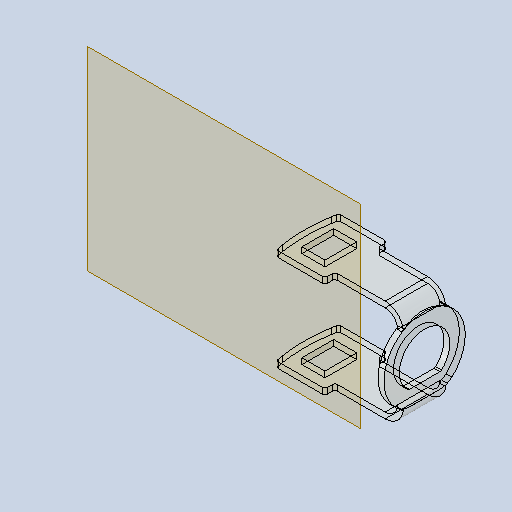
# Autodesk Inventor part: Part3 - Gearbox
Saved by Autodesk Inventor 2023 (Build 270158000, 158)
## iProperties
Created: 2020-10-26
Part Number: Part3 - Gearbox
Material: Glass
Document SubType Name: Modeling
Designer: Niels
Density: 2.18 g/cm^3
Appearance: Clear
MAAT: ØLxBxD
Author: Niels
Autodesk Inventor part; units mm, degrees
ref_plane "YZ Plane" through (0, 0, 0) normal (1, 0, 0) x (0, 1, 0)
ref_plane "XZ Plane" through (0, 0, 0) normal (0, 1, 0) x (-1, 0, 0)
ref_plane "XY Plane" through (0, 0, 0) normal (0, 0, 1) x (1, 0, 0)
ref_plane "Work Plane1" through (0, 0, -6) normal (0, 0, 1) x (1, 0, 0)
sketch "Sketch2" plane through (0, 0, -6) normal (0, 0, 1) x (1, 0, 0)
  line L0 (-0.1721, 1.3319) -> (-0.1721, -0.6681) projected
  line L1 (-0.1721, -0.6681) -> (-1.1721, -0.6681) projected
  line L2 (-1.1721, -0.6681) -> (-1.1721, -1.1681) projected
  line L3 (-1.1721, -1.1681) -> (0.1026, -1.1681) projected
  line L4 (0.1026, -1.1681) -> (1.1279, 1.3319) projected
  line L5 (-0.1721, 1.3319) -> (1.1279, 1.3319) projected
  line L6 (21.2279, 14.4069) -> (21.2279, 6.7069) projected
  line L7 (22.1279, 8.9819) -> (22.1279, 10.9819) projected
  line L8 (-1.5666, 1.1673) -> (16.9443, 1.1673)
  arc A0 (16.9443, 1.1673) -> (19.3523, 3.5752) centre (16.9443, 3.5752) ccw
  line L9 (19.3523, 3.5752) -> (19.3523, 9.9819)
  line L10 (20.5023, 9.9819) -> (20.5023, 3.5752)
  arc A1 (16.9443, 0.0173) -> (20.5023, 3.5752) centre (16.9443, 3.5752) ccw
  line L11 (16.9443, 0.0173) -> (-1.5666, 0.0173)
  line L12 (-1.5666, 0.0173) -> (-1.5666, 1.1673)
  line L13 (20.5023, 9.9819) -> (19.3523, 9.9819)
  line L14 (-1.5666, 18.7964) -> (16.9443, 18.7964)
  arc A2 (19.3523, 16.3885) -> (16.9443, 18.7964) centre (16.9443, 16.3885) ccw
  line L15 (19.3523, 16.3885) -> (19.3523, 9.9819)
  line L16 (20.5023, 9.9819) -> (20.5023, 16.3885)
  arc A3 (20.5023, 16.3885) -> (16.9443, 19.9464) centre (16.9443, 16.3885) ccw
  line L17 (16.9443, 19.9464) -> (-1.5666, 19.9464)
  line L18 (-1.5666, 19.9464) -> (-1.5666, 18.7964)
  point P0 (0, 0)
  point P1 (22.1279, 9.9819)
  dimension "d1" = 1.15
  dimension "d2" = 0.7257
  constraints: 22 end point, 8 point on circle, 7 symmetric about line, 4 centre point, 2 horizontal, 2 tangent, 1 horizontal alignment, 1 midpoint, 1 parallel, 1 vertical, 4 other
  measures "d1" radial gap between concentric circles of A0 A1
  measures "d2" distance between parallel lines of L6 L10
extrude "Extrusion1" add sketch "Sketch2" along normal mid plane 8.3 contours L8 L4 L11 L0 | L0 L11 L12 L8 | L8 A0 L9 L13 L10 A1 L11 L4 | L15 A2 L14 L18 L17 A3 L16 L13
sketch "Sketch3" plane through (20.5023, 3.5752, -1.85) normal (1, 0, 0) x (0, 0, -1)
  line L0 (1.1743, 2.6316) -> (7.1257, 2.6316) projected
  line L1 (1.1743, 2.6316) -> (7.1257, 2.6316) projected
  arc A0 (0.838, 2.7615) -> (1.1743, 2.6316) centre (1.1743, 3.1316) ccw projected
  arc A1 (7.462, 2.7615) -> (0.838, 2.7615) centre (4.15, 6.4066) ccw projected
  arc A2 (7.1257, 2.6316) -> (7.462, 2.7615) centre (7.1257, 3.1316) ccw projected
  line L2 (1.1743, 2.6316) -> (7.1257, 2.6316) projected
  arc A3 (-1.1794, 0.5412) -> (1.1743, -0.3684) centre (1.1743, 3.1316) ccw
  arc A4 (9.4794, 0.5412) -> (-1.1794, 0.5412) centre (4.15, 6.4066) ccw
  arc A5 (7.1257, -0.3684) -> (9.4794, 0.5412) centre (7.1257, 3.1316) ccw
  line L3 (7.1257, -0.3684) -> (1.1743, -0.3684)
  point P0 (-1.85, -3.5752)
  dimension "d5" = 3
  constraints: 6 point on circle, 3 centre point, 2 end point, 1 horizontal, 2 other
  measures "d5" radial gap between concentric circles of A1 A4
extrude "Extrusion2" add sketch "Sketch3" against normal blind 1.15
sketch "Sketch4" plane through (20.5023, 9.9819, -6) normal (1, 0, 0) x (0, 0, -1)
  line L0 (-2.9757, -3.775) -> (2.9757, -3.775) projected
  line L1 (-2.9757, -3.775) -> (2.9757, -3.775) projected
  arc A0 (-3.312, -3.6451) -> (-2.9757, -3.775) centre (-2.9757, -3.275) ccw projected
  arc A1 (3.312, -3.6451) -> (-3.312, -3.6451) centre (0, 0) ccw projected
  arc A2 (2.9757, -3.775) -> (3.312, -3.6451) centre (2.9757, -3.275) ccw projected
  point P0 (-6, -9.9819)
extrude "Extrusion3" cut sketch "Sketch4" against normal blind 1.5
fillet "Fillet1" radius 0.5 4 edges at (19.9253, 3.4097, -1.85) (19.9253, 3.4097, -10.15) (19.9189, 16.7334, -10.15) (19.9189, 16.7334, -1.85)
sketch "Sketch5" plane through (-1.5666, 0.0173, -1.85) normal (0, -1, 0) x (1, 0, 0)
  line L0 (1.3946, -7.15) -> (1.3946, -1.15) projected
  line L1 (1.3946, -1.15) -> (1.3946, -7.15) projected
  line L2 (1.6693, -1.15) -> (2.6946, -1.15) projected
  line L3 (1.6693, -1.15) -> (1.6693, -7.15) projected
  line L4 (1.6693, -7.15) -> (2.6946, -7.15) projected
  line L5 (2.6946, -1.15) -> (2.6946, -7.15) projected
  line L6 (1.1946, -7.25) -> (5.6946, -7.25)
  line L7 (5.6946, -7.25) -> (5.6946, -1.05)
  line L8 (5.6946, -1.05) -> (1.1946, -1.05)
  line L9 (1.1946, -1.05) -> (1.1946, -7.25)
  point P0 (1.5666, 1.85)
  dimension "d12" = 0.1
  dimension "d13" = 0.1
  dimension "d14" = 3
  dimension "d15" = 0.2
  constraints: 8 end point, 2 parallel, 1 horizontal, 1 perpendicular
  measures "d12" distance between parallel lines of L2 L8
  measures "d13" distance between parallel lines of L6 L4
  measures "d14" distance between parallel lines of L7 L5
  measures "d15" distance between parallel lines of L0 L9
extrude "Extrusion4" cut sketch "Sketch5" against normal blind 22.75 contours L2 L5 L4 L3 | L9 L8 L7 L6
sketch "Sketch6" plane through (-1.5666, 0.0173, -1.85) normal (0, -1, 0) x (1, 0, 0)
  line L0 (-0.3816, -10.25) -> (8.1946, -10.25)
  line L1 (8.6946, -9.75) -> (8.6946, 1.45)
  line L2 (8.1946, 1.95) -> (-0.3799, 1.95)
  line L3 (-0.8749, -9.8319) -> (-0.9996, -9.0812)
  line L4 (-1.0196, 0.6268) -> (-0.8734, 1.5299)
  line L5 (1.1946, -1.05) -> (5.6946, -1.05) projected
  line L6 (5.6946, -7.25) -> (1.1946, -7.25) projected
  line L7 (5.6946, -1.05) -> (5.6946, -7.25) projected
  line L8 (1.1946, -7.25) -> (1.1946, -1.05) projected
  arc A0 (-1.0196, 0.6268) -> (-0.9996, -9.0812) centre (28.5951, -4.1661) ccw
  arc A1 (-0.8749, -9.8319) -> (-0.3816, -10.25) centre (-0.3816, -9.75) ccw
  arc A2 (-0.3799, 1.95) -> (-0.8734, 1.5299) centre (-0.3799, 1.45) ccw
  arc A3 (8.6946, 1.45) -> (8.1946, 1.95) centre (8.1946, 1.45) ccw
  arc A4 (8.1946, -10.25) -> (8.6946, -9.75) centre (8.1946, -9.75) ccw
  point P0 (1.5666, 1.85)
  point P1 (-0.8054, -10.25)
  point P2 (-0.8054, 1.95)
  point P3 (-1.8054, -4.2289)
  dimension "d18" = 3
  dimension "d19" = 3
  dimension "d20" = 3
  dimension "d21" = 3
  dimension "d22" = 2
  dimension "d23" = 30
  dimension "d24" = 0.5
  constraints: 10 end point, 10 point on circle, 10 tangent, 6 point on line, 5 centre point, 3 equal radius, 1 horizontal, 1 parallel, 1 perpendicular, 1 vertical alignment
  measures "d18" distance between parallel lines of L2 L5
  measures "d19" distance between parallel lines of L0 L6
  measures "d20" distance between parallel lines of L1 L7
  measures "d21" distance from line of point (-1.805, -4.229) L8
  measures "d22" distance from line of L8 point (-0.805, 1.95)
  measures "d23" radius of A0
  measures "d24" radius of A1
extrude "Extrusion5" add sketch "Sketch6" against normal blind 1.15
sketch "Sketch7" plane through (-1.5666, 19.9464, -1.85) normal (0, 1, 0) x (1, 0, 0)
  line L0 (5.6946, 1.05) -> (5.6946, 7.25) projected
  line L1 (5.6946, 7.25) -> (1.1946, 7.25) projected
  line L2 (1.1946, 7.25) -> (1.1946, 1.05) projected
  line L3 (1.1946, 1.05) -> (5.6946, 1.05) projected
  line L4 (18.5109, 8.3) -> (8.6946, 8.3) projected
  line L5 (18.5109, 8.3) -> (18.5109, 0) projected
  line L6 (8.6946, 0) -> (18.5109, 0) projected
  line L7 (8.6946, -1.45) -> (8.6946, 0) projected
  arc A0 (8.1946, -1.95) -> (8.6946, -1.45) centre (8.1946, -1.45) ccw projected
  line L8 (-0.3799, -1.95) -> (8.1946, -1.95) projected
  arc A1 (-0.8734, -1.5299) -> (-0.3799, -1.95) centre (-0.3799, -1.45) ccw projected
  line L9 (-1.0196, -0.6268) -> (-0.8734, -1.5299) projected
  arc A2 (-0.9996, 9.0812) -> (-1.0196, -0.6268) centre (28.5951, 4.1661) ccw projected
  line L10 (-0.8749, 9.8319) -> (-0.9996, 9.0812) projected
  arc A3 (-0.3816, 10.25) -> (-0.8749, 9.8319) centre (-0.3816, 9.75) ccw projected
  line L11 (8.1946, 10.25) -> (-0.3816, 10.25) projected
  arc A4 (8.6946, 9.75) -> (8.1946, 10.25) centre (8.1946, 9.75) ccw projected
  line L12 (8.6946, 8.3) -> (8.6946, 9.75) projected
  point P0 (1.5666, -1.85)
extrude "Extrusion6" add sketch "Sketch7" against normal blind 1.15
fillet "Fillet2" radius 0.5 4 edges at (7.1279, 19.3714, -1.85) (7.1279, 0.5923, -1.85) (7.1279, 19.3714, -10.15) (7.1279, 0.5923, -10.15)
body "Solid1"
